Autodesk Inventor part; units mm, degrees
(part 2 of 3)
sketch "スケッチ2" plane through (0, 0, 4) normal (0, 0, 1) x (1, 0, 0)
  arc A0 (149.035, 132.768) -> (148.9038, 132.247) centre (154.985, 130.9929) ccw projected
  arc A1 (148.9038, 132.247) -> (148.0962, 132.247) centre (148.5, 105) ccw projected
  arc A2 (148.0962, 132.247) -> (147.965, 132.768) centre (142.015, 130.9929) ccw projected
  arc A3 (147.965, 132.768) -> (147.7093, 133.5027) centre (139.7412, 130.3182) ccw projected
  arc A4 (147.7093, 133.5027) -> (147.2659, 134.4742) centre (137.4161, 129.3913) ccw projected
  arc A5 (147.2659, 134.4742) -> (146.4842, 134.431) centre (148.5, 105) ccw projected
  arc A6 (146.4842, 134.431) -> (146.1503, 133.4167) centre (156.8334, 130.4626) ccw projected
  arc A7 (146.1503, 133.4167) -> (145.977, 132.6583) centre (154.4205, 131.128) ccw projected
  arc A8 (145.977, 132.6583) -> (145.904, 132.1261) centre (152.0862, 131.5485) ccw projected
  arc A9 (145.904, 132.1261) -> (145.1012, 132.0372) centre (148.5, 105) ccw projected
  arc A10 (145.1012, 132.0372) -> (144.9135, 132.5406) centre (139.195, 130.1217) ccw projected
  arc A11 (144.9135, 132.5406) -> (144.5786, 133.2427) centre (137.0091, 129.201) ccw projected
  arc A12 (144.5786, 133.2427) -> (144.031, 134.1595) centre (134.8001, 128.024) ccw projected
  arc A13 (144.031, 134.1595) -> (143.2588, 134.0307) centre (148.5, 105) ccw projected
  arc A14 (143.2588, 134.0307) -> (143.0385, 132.9857) centre (153.9817, 131.2248) ccw projected
  arc A15 (143.0385, 132.9857) -> (142.9497, 132.2129) centre (151.5102, 131.6208) ccw projected
  arc A16 (142.9497, 132.2129) -> (142.9356, 131.6758) centre (149.1439, 131.7819) ccw projected
  arc A17 (142.9356, 131.6758) -> (142.1475, 131.4992) centre (148.5, 105) ccw projected
  arc A18 (142.1475, 131.4992) -> (141.9056, 131.9789) centre (136.4879, 128.9456) ccw projected
  arc A19 (141.9056, 131.9789) -> (141.4955, 132.6399) centre (134.4166, 127.79) ccw projected
  arc A20 (141.4955, 132.6399) -> (140.8503, 133.4909) centre (132.3504, 126.3771) ccw projected
  arc A21 (140.8503, 133.4909) -> (140.097, 133.2779) centre (148.5, 105) ccw projected
  arc A22 (140.097, 133.2779) -> (139.993, 132.2151) centre (151.0635, 131.6687) ccw projected
  arc A23 (139.993, 132.2151) -> (139.9898, 131.4372) centre (148.5635, 131.7903) ccw projected
  arc A24 (139.9898, 131.4372) -> (140.0349, 130.9018) centre (146.1937, 131.6901) ccw projected
  arc A25 (140.0349, 130.9018) -> (139.271, 130.6396) centre (148.5, 105) ccw projected
  arc A26 (139.271, 130.6396) -> (138.9777, 131.0897) centre (133.9266, 127.4788) ccw projected
  arc A27 (138.9777, 131.0897) -> (138.4974, 131.7016) centre (131.995, 126.1024) ccw projected
  arc A28 (138.4974, 131.7016) -> (137.7625, 132.4765) centre (130.0968, 124.4708) ccw projected
  arc A29 (137.7625, 132.4765) -> (137.0372, 132.1819) centre (148.5, 105) ccw projected
  arc A30 (137.0372, 132.1819) -> (137.0508, 131.1141) centre (148.1142, 131.7888) ccw projected
  arc A31 (137.0508, 131.1141) -> (137.1331, 130.3405) centre (145.6159, 131.6347) ccw projected
  arc A32 (137.1331, 130.3405) -> (137.2368, 129.8134) centre (143.2716, 131.2744) ccw projected
  arc A33 (137.2368, 129.8134) -> (136.5064, 129.4687) centre (148.5, 105) ccw projected
  arc A34 (136.5064, 129.4687) -> (136.1654, 129.8839) centre (131.5421, 125.7392) ccw projected
  arc A35 (136.1654, 129.8839) -> (135.6207, 130.4392) centre (129.7737, 124.1586) ccw projected
  arc A36 (135.6207, 130.4392) -> (134.8051, 131.1285) centre (128.0665, 122.3281) ccw projected
  arc A37 (134.8051, 131.1285) -> (134.1165, 130.7559) centre (148.5, 105) ccw projected
  arc A38 (134.1165, 130.7559) -> (134.2475, 129.6961) centre (145.1695, 131.5838) ccw projected
  arc A39 (134.2475, 129.6961) -> (134.4144, 128.9363) centre (142.7034, 131.1558) ccw projected
  arc A40 (134.4144, 128.9363) -> (134.5755, 128.4237) centre (140.4129, 130.5398) ccw projected
  arc A41 (134.5755, 128.4237) -> (133.8875, 128.0008) centre (148.5, 105) ccw projected
  arc A42 (133.8875, 128.0008) -> (133.5029, 128.3759) centre (129.3636, 123.7478) ccw projected
  arc A43 (133.5029, 128.3759) -> (132.9003, 128.868) centre (127.7797, 121.9823) ccw projected
  arc A44 (132.9003, 128.868) -> (132.0138, 129.4634) centre (126.2843, 119.9751) ccw projected
  arc A45 (132.0138, 129.4634) -> (131.3705, 129.0173) centre (148.5, 105) ccw projected
  arc A46 (131.3705, 129.0173) -> (131.6172, 127.9783) centre (142.2653, 131.0561) ccw projected
  arc A47 (131.6172, 127.9783) -> (131.8667, 127.2415) centre (139.8612, 130.3594) ccw projected
  arc A48 (131.8667, 127.2415) -> (132.0832, 126.7498) centre (137.6524, 129.4952) ccw projected
  arc A49 (132.0832, 126.7498) -> (131.4459, 126.2537) centre (148.5, 105) ccw projected
  arc A50 (131.4459, 126.2537) -> (131.0223, 126.5843) centre (127.4173, 121.5289) ccw projected
  arc A51 (131.0223, 126.5843) -> (130.3693, 127.007) centre (126.0373, 119.5998) ccw projected
  arc A52 (130.3693, 127.007) -> (129.4227, 127.5013) centre (124.7718, 117.4403) ccw projected
  arc A53 (129.4227, 127.5013) -> (128.8323, 126.9871) centre (148.5, 105) ccw projected
  arc A54 (128.8323, 126.9871) -> (129.1919, 125.9816) centre (139.4368, 130.2121) ccw projected
  arc A55 (129.1919, 125.9816) -> (129.5209, 125.2767) centre (137.1239, 129.2551) ccw projected
  arc A56 (129.5209, 125.2767) -> (129.7902, 124.8118) centre (135.0236, 128.1532) ccw projected
  arc A57 (129.7902, 124.8118) -> (129.2113, 124.2486) centre (148.5, 105) ccw projected
  arc A58 (129.2113, 124.2486) -> (128.754, 124.5306) centre (125.727, 119.1093) ccw projected
  arc A59 (128.754, 124.5306) -> (128.0584, 124.8789) centre (124.5675, 117.0401) ccw projected
  arc A60 (128.0584, 124.8789) -> (127.0632, 125.2661) centre (123.5472, 114.7545) ccw projected
  arc A61 (127.0632, 125.2661) -> (126.5329, 124.69) centre (148.5, 105) ccw projected
  arc A62 (126.5329, 124.69) -> (127.0009, 123.7302) centre (136.7182, 129.062) ccw projected
  arc A63 (127.0009, 123.7302) -> (127.4055, 123.0658) centre (134.5247, 127.8564) ccw projected
  arc A64 (127.4055, 123.0658) -> (127.7243, 122.6333) centre (132.5583, 126.5301) ccw projected
  arc A65 (127.7243, 122.6333) -> (127.2109, 122.0099) centre (148.5, 105) ccw projected
  arc A66 (127.2109, 122.0099) -> (126.7253, 122.2398) centre (124.313, 116.5184) ccw projected
  arc A67 (126.7253, 122.2398) -> (125.9956, 122.5095) centre (123.3883, 114.3343) ccw projected
  arc A68 (125.9956, 122.5095) -> (124.9639, 122.7848) centre (122.6256, 111.9503) ccw projected
  arc A69 (124.9639, 122.7848) -> (124.5002, 122.154) centre (148.5, 105) ccw projected
  arc A70 (124.5002, 122.154) -> (125.0709, 121.2514) centre (134.1427, 127.6199) ccw projected
  arc A71 (125.0709, 121.2514) -> (125.5462, 120.6355) centre (132.0951, 126.1803) ccw projected
  arc A72 (125.5462, 120.6355) -> (125.9106, 120.2408) centre (130.2866, 124.6457) ccw projected
  arc A73 (125.9106, 120.2408) -> (125.4688, 119.5646) centre (148.5, 105) ccw projected
  arc A74 (125.4688, 119.5646) -> (124.9609, 119.7398) centre (123.1927, 113.7878) ccw projected
  arc A75 (124.9609, 119.7398) -> (124.206, 119.9276) centre (122.5139, 111.5151) ccw projected
  arc A76 (124.206, 119.9276) -> (123.1502, 120.0877) centre (122.0181, 109.0617) ccw projected
  arc A77 (123.1502, 120.0877) -> (122.7588, 119.4097) centre (148.5, 105) ccw projected
  arc A78 (122.7588, 119.4097) -> (123.4253, 118.5754) centre (131.7415, 125.9032) ccw projected
  arc A79 (123.4253, 118.5754) -> (123.9655, 118.0155) centre (129.8647, 124.2471) ccw projected
  arc A80 (123.9655, 118.0155) -> (124.3711, 117.6632) centre (128.2359, 122.5229) ccw projected
  arc A81 (124.3711, 117.6632) -> (124.0064, 116.9426) centre (148.5, 105) ccw projected
  arc A82 (124.0064, 116.9426) -> (123.4823, 117.0608) centre (122.3796, 110.9504) ccw projected
  arc A83 (123.4823, 117.0608) -> (122.7113, 117.1645) centre (121.9549, 108.6169) ccw projected
  arc A84 (122.7113, 117.1645) -> (121.6443, 117.2075) centre (121.732, 106.1238) ccw projected
  arc A85 (121.6443, 117.2075) -> (121.3298, 116.4905) centre (148.5, 105) ccw projected
  arc A86 (121.3298, 116.4905) -> (122.0841, 115.7346) centre (129.5437, 123.9327) ccw projected
  arc A87 (122.0841, 115.7346) -> (122.6825, 115.2375) centre (127.8604, 122.0802) ccw projected
  arc A88 (122.6825, 115.2375) -> (123.1245, 114.932) centre (126.4313, 120.1873) ccw projected
  arc A89 (123.1245, 114.932) -> (122.8413, 114.1756) centre (148.5, 105) ccw projected
  arc A90 (122.8413, 114.1756) -> (122.3074, 114.2355) centre (121.8835, 108.0408) ccw projected
  arc A91 (122.3074, 114.2355) -> (121.5297, 114.2537) centre (121.7181, 105.6748) ccw projected
  arc A92 (121.5297, 114.2537) -> (120.4644, 114.179) centre (121.7708, 103.1723) ccw projected
  arc A93 (120.4644, 114.179) -> (120.2307, 113.4318) centre (148.5, 105) ccw projected
  arc A94 (120.2307, 113.4318) -> (121.0636, 112.7635) centre (127.576, 121.7325) ccw projected
  arc A95 (121.0636, 112.7635) -> (121.713, 112.3353) centre (126.1067, 119.7061) ccw projected
  arc A96 (121.713, 112.3353) -> (122.1859, 112.0802) centre (124.8945, 117.6674) ccw projected
  arc A97 (122.1859, 112.0802) -> (121.9876, 111.2973) centre (148.5, 105) ccw projected
  arc A98 (121.9876, 111.2973) -> (121.4504, 111.298) centre (121.7106, 105.0943) ccw projected
  arc A99 (121.4504, 111.298) -> (120.6754, 111.2305) centre (121.8064, 102.7244) ccw projected
  arc A100 (120.6754, 111.2305) -> (119.6248, 111.0392) centre (122.1341, 100.243) ccw projected
  arc A101 (119.6248, 111.0392) -> (119.4747, 110.2708) centre (148.5, 105) ccw projected
  arc A102 (119.4747, 110.2708) -> (120.376, 109.6981) centre (125.8623, 119.3291) ccw projected
  arc A103 (120.376, 109.6981) -> (121.0687, 109.344) centre (124.6249, 117.1534) ccw projected
  arc A104 (121.0687, 109.344) -> (121.5667, 109.1425) centre (123.6442, 114.9937) ccw projected
  arc A105 (121.5667, 109.1425) -> (121.4558, 108.3425) centre (148.5, 105) ccw projected
  arc A106 (121.4558, 108.3425) -> (120.9217, 108.2841) centre (121.8628, 102.1467) ccw projected
  arc A107 (120.9217, 108.2841) -> (120.1588, 108.1318) centre (122.2187, 99.8017) ccw projected
  arc A108 (120.1588, 108.1318) -> (119.1357, 107.826) centre (122.8174, 97.3714) ccw projected
  arc A109 (119.1357, 107.826) -> (119.071, 107.0458) centre (148.5, 105) ccw projected
  arc A110 (119.071, 107.0458) -> (120.0299, 106.5757) centre (124.4233, 116.7518) ccw projected
  arc A111 (120.0299, 106.5757) -> (120.7573, 106.2999) centre (123.4328, 114.4531) ccw projected
  arc A112 (120.7573, 106.2999) -> (121.2745, 106.1544) centre (122.6957, 112.1987) ccw projected
  arc A113 (121.2745, 106.1544) -> (121.2522, 105.3471) centre (148.5, 105) ccw projected
  arc A114 (121.2522, 105.3471) -> (120.7278, 105.2303) centre (122.3383, 99.2337) ccw projected
  arc A115 (120.7278, 105.2303) -> (119.9863, 104.995) centre (122.9501, 96.9421) ccw projected
  arc A116 (119.9863, 104.995) -> (119.003, 104.5785) centre (123.8125, 94.5924) ccw projected
  arc A117 (119.003, 104.5785) -> (119.0246, 103.7959) centre (148.5, 105) ccw projected
  arc A118 (119.0246, 103.7959) -> (120.0294, 103.4342) centre (123.2767, 114.0318) ccw projected
  arc A119 (120.0294, 103.4342) -> (120.7827, 103.2401) centre (122.545, 111.6382) ccw projected
  arc A120 (120.7827, 103.2401) -> (121.3127, 103.1524) centre (122.0604, 109.3163) ccw projected
  arc A121 (121.3127, 103.1524) -> (121.3794, 102.3475) centre (148.5, 105) ccw projected
  arc A122 (121.3794, 102.3475) -> (120.871, 102.1738) centre (123.1315, 96.3907) ccw projected
  arc A123 (120.871, 102.1738) -> (120.1599, 101.8583) centre (123.9916, 94.1803) ccw projected
  arc A124 (120.1599, 101.8583) -> (119.2284, 101.3362) centre (125.1073, 91.9397) ccw projected
  arc A125 (119.2284, 101.3362) -> (119.3359, 100.5607) centre (148.5, 105) ccw projected
  arc A126 (119.3359, 100.5607) -> (120.3744, 100.3117) centre (122.4362, 111.2023) ccw projected
  arc A127 (120.3744, 100.3117) -> (121.1445, 100.2017) centre (121.9723, 108.7426) ccw projected
  arc A128 (121.1445, 100.2017) -> (121.681, 100.1728) centre (121.746, 106.3816) ccw projected
  arc A129 (121.681, 100.1728) -> (121.8358, 99.3801) centre (148.5, 105) ccw projected
  arc A130 (121.8358, 99.3801) -> (121.3496, 99.1515) centre (124.2325, 93.6522) ccw projected
  arc A131 (121.3496, 99.1515) -> (120.6776, 98.7597) centre (125.3306, 91.5499) ccw projected
  arc A132 (120.6776, 98.7597) -> (119.8091, 98.1383) centre (126.686, 89.4456) ccw projected
  arc A133 (119.8091, 98.1383) -> (120.0013, 97.3793) centre (148.5, 105) ccw projected
  arc A134 (120.0013, 97.3793) -> (121.0608, 97.2461) centre (121.9121, 108.2974) ccw projected
  arc A135 (121.0608, 97.2461) -> (121.8384, 97.2214) centre (121.7216, 105.8016) ccw projected
  arc A136 (121.8384, 97.2214) -> (122.3748, 97.2518) centre (121.7564, 103.43) ccw projected
  arc A137 (122.3748, 97.2518) -> (122.6159, 96.481) centre (148.5, 105) ccw projected
  arc A138 (122.6159, 96.481) -> (122.1578, 96.2002) centre (125.6281, 91.0515) ccw projected
  arc A139 (122.1578, 96.2002) -> (121.5329, 95.7369) centre (126.9509, 89.0827) ccw projected
  arc A140 (121.5329, 95.7369) -> (120.7381, 95.0237) centre (128.5295, 87.1403) ccw projected
  arc A141 (120.7381, 95.0237) -> (121.0126, 94.2905) centre (148.5, 105) ccw projected
  arc A142 (121.0126, 94.2905) -> (122.0804, 94.2747) centre (121.7107, 105.3525) ccw projected
  arc A143 (122.0804, 94.2747) -> (122.8559, 94.3357) centre (121.7959, 102.8509) ccw projected
  arc A144 (122.8559, 94.3357) -> (123.3857, 94.4248) centre (122.0915, 100.4975) ccw projected
  arc A145 (123.3857, 94.4248) -> (123.7101, 93.6852) centre (148.5, 105) ccw projected
  arc A146 (123.7101, 93.6852) -> (123.2857, 93.3558) centre (127.3014, 88.62) ccw projected
  arc A147 (123.2857, 93.3558) -> (122.7156, 92.8265) centre (128.8327, 86.8087) ccw projected
  arc A148 (122.7156, 92.8265) -> (122.0041, 92.0302) centre (130.6154, 85.0518) ccw projected
  arc A149 (122.0041, 92.0302) -> (122.3576, 91.3317) centre (148.5, 105) ccw projected
  arc A150 (122.3576, 91.3317) -> (123.4206, 91.4334) centre (121.8345, 102.4033) ccw projected
  arc A151 (123.4206, 91.4334) -> (124.1847, 91.5793) centre (122.1944, 99.9263) ccw projected
  arc A152 (124.1847, 91.5793) -> (124.7015, 91.7262) centre (122.7471, 97.6197) ccw projected
  arc A153 (124.7015, 91.7262) -> (125.1053, 91.0268) centre (148.5, 105) ccw projected
  arc A154 (125.1053, 91.0268) -> (124.7197, 90.6527) centre (129.232, 86.3874) ccw projected
  arc A155 (124.7197, 90.6527) -> (124.2113, 90.0639) centre (130.9532, 84.7555) ccw projected
  arc A156 (124.2113, 90.0639) -> (123.5917, 89.1942) centre (132.9185, 83.2054) ccw projected
  arc A157 (123.5917, 89.1942) -> (124.0199, 88.5387) centre (148.5, 105) ccw projected
  arc A158 (124.0199, 88.5387) -> (125.0653, 88.7568) centre (122.282, 99.4856) ccw projected
  arc A159 (125.0653, 88.7568) -> (125.8087, 88.9859) centre (122.9122, 97.0632) ccw projected
  arc A160 (125.8087, 88.9859) -> (126.3062, 89.1887) centre (123.7152, 94.8315) ccw projected
  arc A161 (126.3062, 89.1887) -> (126.7845, 88.538) centre (148.5, 105) ccw projected
  arc A162 (126.7845, 88.538) -> (126.4424, 88.1237) centre (131.3965, 84.3808) ccw projected
  arc A163 (126.4424, 88.1237) -> (126.0018, 87.4826) centre (133.2868, 82.9481) ccw projected
  arc A164 (126.0018, 87.4826) -> (125.4816, 86.55) centre (135.4106, 81.6236) ccw projected
  arc A165 (125.4816, 86.55) -> (125.9793, 85.9456) centre (148.5, 105) ccw projected
  arc A166 (125.9793, 85.9456) -> (126.9944, 86.2773) centre (123.0478, 96.6349) ccw projected
  arc A167 (126.9944, 86.2773) -> (127.7081, 86.5869) centre (123.9406, 94.2966) ccw projected
  arc A168 (127.7081, 86.5869) -> (128.1802, 86.8432) centre (124.9843, 92.1667) ccw projected
  arc A169 (128.1802, 86.8432) -> (128.7272, 86.249) centre (148.5, 105) ccw projected
  arc A170 (128.7272, 86.249) -> (128.4328, 85.7996) centre (133.7686, 82.6244) ccw projected
  arc A171 (128.4328, 85.7996) -> (128.0654, 85.1139) centre (135.805, 81.4084) ccw projected
  arc A172 (128.0654, 85.1139) -> (127.651, 84.1297) centre (138.0617, 80.3255) ccw projected
  arc A173 (127.651, 84.1297) -> (128.2121, 83.5838) centre (148.5, 105) ccw projected
  arc A174 (128.2121, 83.5838) -> (129.1845, 84.0252) centre (124.1225, 93.8857) ccw projected
  arc A175 (129.1845, 84.0252) -> (129.8599, 84.4113) centre (125.2672, 91.6598) ccw projected
  arc A176 (129.8599, 84.4113) -> (130.3009, 84.7181) centre (126.5388, 89.6576) ccw projected
  arc A177 (130.3009, 84.7181) -> (130.91, 84.1876) centre (148.5, 105) ccw projected
  arc A178 (130.91, 84.1876) -> (130.6668, 83.7086) centre (136.3195, 81.1396) ccw projected
  arc A179 (130.6668, 83.7086) -> (130.377, 82.9867) centre (138.4773, 80.155) ccw projected
  arc A180 (130.377, 82.9867) -> (130.0734, 81.9628) centre (140.8394, 79.3269) ccw projected
  arc A181 (130.0734, 81.9628) -> (130.6912, 81.482) centre (148.5, 105) ccw projected
  arc A182 (130.6912, 81.482) -> (131.6092, 82.0276) centre (125.4931, 91.2715) ccw projected
  arc A183 (131.6092, 82.0276) -> (132.2379, 82.4857) centre (126.8757, 89.1849) ccw projected
  arc A184 (132.2379, 82.4857) -> (132.6426, 82.8391) centre (128.3599, 87.3348) ccw projected
  arc A185 (132.6426, 82.8391) -> (133.3063, 82.3789) centre (148.5, 105) ccw projected
  arc A186 (133.3063, 82.3789) -> (133.1172, 81.876) centre (139.0183, 79.9445) ccw projected
  arc A187 (133.1172, 81.876) -> (132.9087, 81.1266) centre (141.2713, 79.2032) ccw projected
  arc A188 (132.9087, 81.1266) -> (132.7195, 80.0756) centre (143.7101, 78.64) ccw projected
  arc A189 (132.7195, 80.0756) -> (133.3865, 79.6656) centre (148.5, 105) ccw projected
  arc A190 (133.3865, 79.6656) -> (134.2388, 80.3089) centre (127.143, 88.8238) ccw projected
  arc A191 (134.2388, 80.3089) -> (134.8134, 80.8334) centre (128.7467, 86.9021) ccw projected
  arc A192 (134.8134, 80.8334) -> (135.1767, 81.2292) centre (130.4254, 85.2265) ccw projected
  arc A193 (135.1767, 81.2292) -> (135.887, 80.8448) centre (148.5, 105) ccw projected
  arc A194 (135.887, 80.8448) -> (135.7544, 80.3241) centre (141.8321, 79.0535) ccw projected
  arc A195 (135.7544, 80.3241) -> (135.6296, 79.5563) centre (144.153, 78.5646) ccw projected
  arc A196 (135.6296, 79.5563) -> (135.5572, 78.4909) centre (146.639, 78.2731) ccw projected
  arc A197 (135.5572, 78.4909) -> (136.2652, 78.1567) centre (148.5, 105) ccw projected
  arc A198 (136.2652, 78.1567) -> (137.0416, 78.8899) centre (129.0521, 86.5726) ccw projected
  arc A199 (137.0416, 78.8899) -> (137.555, 79.4744) centre (130.8575, 84.8389) ccw projected
  arc A200 (137.555, 79.4744) -> (137.8726, 79.9078) centre (132.7104, 83.3581) ccw projected
  arc A201 (137.8726, 79.9078) -> (138.6208, 79.6038) centre (148.5, 105) ccw projected
  arc A202 (138.6208, 79.6038) -> (138.5463, 79.0718) centre (144.7269, 78.4774) ccw projected
  arc A203 (138.5463, 79.0718) -> (138.5067, 78.2949) centre (147.0875, 78.2468) ccw projected
  arc A204 (138.5067, 78.2949) -> (138.552, 77.228) centre (149.5905, 78.2306) ccw projected
  arc A205 (138.552, 77.228) -> (139.2925, 76.9737) centre (148.5, 105) ccw projected
  arc A206 (139.2925, 76.9737) -> (139.9835, 77.7879) centre (131.1973, 84.545) ccw projected
  arc A207 (139.9835, 77.7879) -> (140.4294, 78.4253) centre (133.1825, 83.0204) ccw projected
  arc A208 (140.4294, 78.4253) -> (140.6974, 78.891) centre (135.187, 81.7525) ccw projected
  arc A209 (140.6974, 78.891) -> (141.4746, 78.6712) centre (148.5, 105) ccw projected
  arc A210 (141.4746, 78.6712) -> (141.459, 78.1342) centre (147.6675, 78.2233) ccw projected
  arc A211 (141.459, 78.1342) -> (141.5051, 77.3576) centre (150.0392, 78.2538) ccw projected
  arc A212 (141.5051, 77.3576) -> (141.6675, 76.3021) centre (152.5287, 78.513) ccw projected
  arc A213 (141.6675, 76.3021) -> (142.4315, 76.1309) centre (148.5, 105) ccw projected
  arc A214 (142.4315, 76.1309) -> (143.0287, 77.0162) centre (133.5526, 82.7657) ccw projected
  arc A215 (143.0287, 77.0162) -> (143.4018, 77.6988) centre (135.6934, 81.4688) ccw projected
  arc A216 (143.4018, 77.6988) -> (143.617, 78.1911) centre (137.8252, 80.429) ccw projected
  arc A217 (143.617, 78.1911) -> (144.4136, 78.0581) centre (148.5, 105) ccw projected
  arc A218 (144.4136, 78.0581) -> (144.4572, 77.5227) centre (150.6182, 78.2943) ccw projected
  arc A219 (144.4572, 77.5227) -> (144.5885, 76.7559) centre (152.9721, 78.5855) ccw projected
  arc A220 (144.5885, 76.7559) -> (144.866, 75.7247) centre (155.4181, 79.117) ccw projected
  arc A221 (144.866, 75.7247) -> (145.6441, 75.6386) centre (148.5, 105) ccw projected
  arc A222 (145.6441, 75.6386) -> (146.1404, 76.5841) centre (136.0892, 81.2563) ccw projected
  arc A223 (146.1404, 76.5841) -> (146.4361, 77.3036) centre (138.3598, 80.2028) ccw projected
  arc A224 (146.4361, 77.3036) -> (146.5958, 77.8166) centre (140.593, 79.4039) ccw projected
  arc A225 (146.5958, 77.8166) -> (147.4022, 77.7721) centre (148.5, 105) ccw projected
  arc A226 (147.4022, 77.7721) -> (147.5045, 77.2447) centre (153.5432, 78.6894) ccw projected
  arc A227 (147.5045, 77.2447) -> (147.7193, 76.497) centre (155.8508, 79.2378) ccw projected
  arc A228 (147.7193, 76.497) -> (148.1085, 75.5026) centre (158.2234, 80.0351) ccw projected
  arc A229 (148.1085, 75.5026) -> (148.8915, 75.5026) centre (148.5, 105) ccw projected
  arc A230 (148.8915, 75.5026) -> (149.2807, 76.497) centre (138.7766, 80.0351) ccw projected
  arc A231 (149.2807, 76.497) -> (149.4955, 77.2447) centre (141.1492, 79.2378) ccw projected
  arc A232 (149.4955, 77.2447) -> (149.5978, 77.7721) centre (143.4568, 78.6894) ccw projected
  arc A233 (149.5978, 77.7721) -> (150.4042, 77.8166) centre (148.5, 105) ccw projected
  arc A234 (150.4042, 77.8166) -> (150.5639, 77.3036) centre (156.407, 79.4039) ccw projected
  arc A235 (150.5639, 77.3036) -> (150.8596, 76.5841) centre (158.6402, 80.2028) ccw projected
  arc A236 (150.8596, 76.5841) -> (151.3559, 75.6386) centre (160.9108, 81.2563) ccw projected
  arc A237 (151.3559, 75.6386) -> (152.134, 75.7247) centre (148.5, 105) ccw projected
  arc A238 (152.134, 75.7247) -> (152.4115, 76.7559) centre (141.5819, 79.117) ccw projected
  arc A239 (152.4115, 76.7559) -> (152.5428, 77.5227) centre (144.0279, 78.5855) ccw projected
  arc A240 (152.5428, 77.5227) -> (152.5864, 78.0581) centre (146.3818, 78.2943) ccw projected
  arc A241 (152.5864, 78.0581) -> (153.383, 78.1911) centre (148.5, 105) ccw projected
  arc A242 (153.383, 78.1911) -> (153.5982, 77.6988) centre (159.1748, 80.429) ccw projected
  arc A243 (153.5982, 77.6988) -> (153.9713, 77.0162) centre (161.3066, 81.4688) ccw projected
  arc A244 (153.9713, 77.0162) -> (154.5685, 76.1309) centre (163.4474, 82.7657) ccw projected
  arc A245 (154.5685, 76.1309) -> (155.3325, 76.3021) centre (148.5, 105) ccw projected
  arc A246 (155.3325, 76.3021) -> (155.4949, 77.3576) centre (144.4713, 78.513) ccw projected
  arc A247 (155.4949, 77.3576) -> (155.541, 78.1342) centre (146.9608, 78.2538) ccw projected
  arc A248 (155.541, 78.1342) -> (155.5254, 78.6712) centre (149.3325, 78.2233) ccw projected
  arc A249 (155.5254, 78.6712) -> (156.3026, 78.891) centre (148.5, 105) ccw projected
  arc A250 (156.3026, 78.891) -> (156.5706, 78.4253) centre (161.813, 81.7525) ccw projected
  arc A251 (156.5706, 78.4253) -> (157.0165, 77.7879) centre (163.8175, 83.0204) ccw projected
  arc A252 (157.0165, 77.7879) -> (157.7075, 76.9737) centre (165.8027, 84.545) ccw projected
  arc A253 (157.7075, 76.9737) -> (158.448, 77.228) centre (148.5, 105) ccw projected
  arc A254 (158.448, 77.228) -> (158.4933, 78.2949) centre (147.4095, 78.2306) ccw projected
  arc A255 (158.4933, 78.2949) -> (158.4537, 79.0718) centre (149.9125, 78.2468) ccw projected
  arc A256 (158.4537, 79.0718) -> (158.3792, 79.6038) centre (152.2731, 78.4774) ccw projected
  arc A257 (158.3792, 79.6038) -> (159.1274, 79.9078) centre (148.5, 105) ccw projected
  arc A258 (159.1274, 79.9078) -> (159.445, 79.4744) centre (164.2896, 83.3581) ccw projected
  arc A259 (159.445, 79.4744) -> (159.9584, 78.8899) centre (166.1425, 84.8389) ccw projected
  arc A260 (159.9584, 78.8899) -> (160.7348, 78.1567) centre (167.9479, 86.5726) ccw projected
  arc A261 (160.7348, 78.1567) -> (161.4428, 78.4909) centre (148.5, 105) ccw projected
  arc A262 (161.4428, 78.4909) -> (161.3704, 79.5563) centre (150.361, 78.2731) ccw projected
  arc A263 (161.3704, 79.5563) -> (161.2456, 80.3241) centre (152.847, 78.5646) ccw projected
  arc A264 (161.2456, 80.3241) -> (161.113, 80.8448) centre (155.1679, 79.0535) ccw projected
  arc A265 (161.113, 80.8448) -> (161.8233, 81.2292) centre (148.5, 105) ccw projected
  arc A266 (161.8233, 81.2292) -> (162.1866, 80.8334) centre (166.5746, 85.2265) ccw projected
  arc A267 (162.1866, 80.8334) -> (162.7612, 80.3089) centre (168.2533, 86.9021) ccw projected
  arc A268 (162.7612, 80.3089) -> (163.6135, 79.6656) centre (169.857, 88.8238) ccw projected
  arc A269 (163.6135, 79.6656) -> (164.2805, 80.0756) centre (148.5, 105) ccw projected
  arc A270 (164.2805, 80.0756) -> (164.0913, 81.1266) centre (153.2899, 78.64) ccw projected
  arc A271 (164.0913, 81.1266) -> (163.8828, 81.876) centre (155.7287, 79.2032) ccw projected
  arc A272 (163.8828, 81.876) -> (163.6937, 82.3789) centre (157.9817, 79.9445) ccw projected
  arc A273 (163.6937, 82.3789) -> (164.3574, 82.8391) centre (148.5, 105) ccw projected
  arc A274 (164.3574, 82.8391) -> (164.7621, 82.4857) centre (168.6401, 87.3348) ccw projected
  arc A275 (164.7621, 82.4857) -> (165.3908, 82.0276) centre (170.1243, 89.1849) ccw projected
  arc A276 (165.3908, 82.0276) -> (166.3088, 81.482) centre (171.5069, 91.2715) ccw projected
  arc A277 (166.3088, 81.482) -> (166.9266, 81.9628) centre (148.5, 105) ccw projected
  arc A278 (166.9266, 81.9628) -> (166.623, 82.9867) centre (156.1606, 79.3269) ccw projected
  arc A279 (166.623, 82.9867) -> (166.3332, 83.7086) centre (158.5227, 80.155) ccw projected
  arc A280 (166.3332, 83.7086) -> (166.09, 84.1876) centre (160.6805, 81.1396) ccw projected
  arc A281 (166.09, 84.1876) -> (166.6991, 84.7181) centre (148.5, 105) ccw projected
  arc A282 (166.6991, 84.7181) -> (167.1401, 84.4113) centre (170.4612, 89.6576) ccw projected
  arc A283 (167.1401, 84.4113) -> (167.8155, 84.0252) centre (171.7328, 91.6598) ccw projected
  arc A284 (167.8155, 84.0252) -> (168.7879, 83.5838) centre (172.8775, 93.8857) ccw projected
  arc A285 (168.7879, 83.5838) -> (169.349, 84.1297) centre (148.5, 105) ccw projected
  arc A286 (169.349, 84.1297) -> (168.9346, 85.1139) centre (158.9383, 80.3255) ccw projected
  arc A287 (168.9346, 85.1139) -> (168.5672, 85.7996) centre (161.195, 81.4084) ccw projected
  arc A288 (168.5672, 85.7996) -> (168.2728, 86.249) centre (163.2314, 82.6244) ccw projected
  arc A289 (168.2728, 86.249) -> (168.8198, 86.8432) centre (148.5, 105) ccw projected
  arc A290 (168.8198, 86.8432) -> (169.2919, 86.5869) centre (172.0157, 92.1667) ccw projected
  arc A291 (169.2919, 86.5869) -> (170.0056, 86.2773) centre (173.0594, 94.2966) ccw projected
  arc A292 (170.0056, 86.2773) -> (171.0207, 85.9456) centre (173.9522, 96.6349) ccw projected
  arc A293 (171.0207, 85.9456) -> (171.5184, 86.55) centre (148.5, 105) ccw projected
  arc A294 (171.5184, 86.55) -> (170.9982, 87.4826) centre (161.5894, 81.6236) ccw projected
  arc A295 (170.9982, 87.4826) -> (170.5576, 88.1237) centre (163.7132, 82.9481) ccw projected
  arc A296 (170.5576, 88.1237) -> (170.2155, 88.538) centre (165.6035, 84.3808) ccw projected
  arc A297 (170.2155, 88.538) -> (170.6938, 89.1887) centre (148.5, 105) ccw projected
  arc A298 (170.6938, 89.1887) -> (171.1913, 88.9859) centre (173.2848, 94.8315) ccw projected
  arc A299 (171.1913, 88.9859) -> (171.9347, 88.7568) centre (174.0878, 97.0632) ccw projected
  arc A300 (171.9347, 88.7568) -> (172.9801, 88.5387) centre (174.718, 99.4856) ccw projected
  arc A301 (172.9801, 88.5387) -> (173.4083, 89.1942) centre (148.5, 105) ccw projected
  arc A302 (173.4083, 89.1942) -> (172.7887, 90.0639) centre (164.0815, 83.2054) ccw projected
  arc A303 (172.7887, 90.0639) -> (172.2803, 90.6527) centre (166.0468, 84.7555) ccw projected
  arc A304 (172.2803, 90.6527) -> (171.8947, 91.0268) centre (167.768, 86.3874) ccw projected
  arc A305 (171.8947, 91.0268) -> (172.2985, 91.7262) centre (148.5, 105) ccw projected
  arc A306 (172.2985, 91.7262) -> (172.8153, 91.5793) centre (174.2529, 97.6197) ccw projected
  arc A307 (172.8153, 91.5793) -> (173.5794, 91.4334) centre (174.8056, 99.9263) ccw projected
  arc A308 (173.5794, 91.4334) -> (174.6424, 91.3317) centre (175.1655, 102.4033) ccw projected
  arc A309 (174.6424, 91.3317) -> (174.9959, 92.0302) centre (148.5, 105) ccw projected
  arc A310 (174.9959, 92.0302) -> (174.2844, 92.8265) centre (166.3846, 85.0518) ccw projected
  arc A311 (174.2844, 92.8265) -> (173.7143, 93.3558) centre (168.1673, 86.8087) ccw projected
  arc A312 (173.7143, 93.3558) -> (173.2899, 93.6852) centre (169.6986, 88.62) ccw projected
  arc A313 (173.2899, 93.6852) -> (173.6143, 94.4248) centre (148.5, 105) ccw projected
  arc A314 (173.6143, 94.4248) -> (174.1441, 94.3357) centre (174.9085, 100.4975) ccw projected
  arc A315 (174.1441, 94.3357) -> (174.9196, 94.2747) centre (175.2041, 102.8509) ccw projected
  arc A316 (174.9196, 94.2747) -> (175.9874, 94.2905) centre (175.2893, 105.3525) ccw projected
  arc A317 (175.9874, 94.2905) -> (176.2619, 95.0237) centre (148.5, 105) ccw projected
  arc A318 (176.2619, 95.0237) -> (175.4671, 95.7369) centre (168.4705, 87.1403) ccw projected
  arc A319 (175.4671, 95.7369) -> (174.8422, 96.2002) centre (170.0491, 89.0827) ccw projected
  arc A320 (174.8422, 96.2002) -> (174.3841, 96.481) centre (171.3719, 91.0515) ccw projected
  arc A321 (174.3841, 96.481) -> (174.6252, 97.2518) centre (148.5, 105) ccw projected
  arc A322 (174.6252, 97.2518) -> (175.1616, 97.2214) centre (175.2436, 103.43) ccw projected
  arc A323 (175.1616, 97.2214) -> (175.9392, 97.2461) centre (175.2784, 105.8016) ccw projected
  arc A324 (175.9392, 97.2461) -> (176.9987, 97.3793) centre (175.0879, 108.2974) ccw projected
  arc A325 (176.9987, 97.3793) -> (177.1909, 98.1383) centre (148.5, 105) ccw projected
  arc A326 (177.1909, 98.1383) -> (176.3224, 98.7597) centre (170.314, 89.4456) ccw projected
  arc A327 (176.3224, 98.7597) -> (175.6504, 99.1515) centre (171.6694, 91.5499) ccw projected
  arc A328 (175.6504, 99.1515) -> (175.1642, 99.3801) centre (172.7675, 93.6522) ccw projected
  arc A329 (175.1642, 99.3801) -> (175.319, 100.1728) centre (148.5, 105) ccw projected
  arc A330 (175.319, 100.1728) -> (175.8555, 100.2017) centre (175.254, 106.3816) ccw projected
  arc A331 (175.8555, 100.2017) -> (176.6256, 100.3117) centre (175.0277, 108.7426) ccw projected
  arc A332 (176.6256, 100.3117) -> (177.6641, 100.5607) centre (174.5638, 111.2023) ccw projected
  arc A333 (177.6641, 100.5607) -> (177.7716, 101.3362) centre (148.5, 105) ccw projected
  arc A334 (177.7716, 101.3362) -> (176.8401, 101.8583) centre (171.8927, 91.9397) ccw projected
  arc A335 (176.8401, 101.8583) -> (176.129, 102.1738) centre (173.0084, 94.1803) ccw projected
  arc A336 (176.129, 102.1738) -> (175.6206, 102.3475) centre (173.8685, 96.3907) ccw projected
  arc A337 (175.6206, 102.3475) -> (175.6873, 103.1524) centre (148.5, 105) ccw projected
  arc A338 (175.6873, 103.1524) -> (176.2173, 103.2401) centre (174.9396, 109.3163) ccw projected
  arc A339 (176.2173, 103.2401) -> (176.9706, 103.4342) centre (174.455, 111.6382) ccw projected
  arc A340 (176.9706, 103.4342) -> (177.9754, 103.7959) centre (173.7233, 114.0318) ccw projected
  arc A341 (177.9754, 103.7959) -> (177.997, 104.5785) centre (148.5, 105) ccw projected
  arc A342 (177.997, 104.5785) -> (177.0137, 104.995) centre (173.1875, 94.5924) ccw projected
  arc A343 (177.0137, 104.995) -> (176.2722, 105.2303) centre (174.0499, 96.9421) ccw projected
  arc A344 (176.2722, 105.2303) -> (175.7478, 105.3471) centre (174.6617, 99.2337) ccw projected
  arc A345 (175.7478, 105.3471) -> (175.7255, 106.1544) centre (148.5, 105) ccw projected
  arc A346 (175.7255, 106.1544) -> (176.2427, 106.2999) centre (174.3043, 112.1987) ccw projected
  arc A347 (176.2427, 106.2999) -> (176.9701, 106.5757) centre (173.5672, 114.4531) ccw projected
  arc A348 (176.9701, 106.5757) -> (177.929, 107.0458) centre (172.5767, 116.7518) ccw projected
  arc A349 (177.929, 107.0458) -> (177.8643, 107.826) centre (148.5, 105) ccw projected
  arc A350 (177.8643, 107.826) -> (176.8412, 108.1318) centre (174.1826, 97.3714) ccw projected
  arc A351 (176.8412, 108.1318) -> (176.0783, 108.2841) centre (174.7813, 99.8017) ccw projected
  arc A352 (176.0783, 108.2841) -> (175.5442, 108.3425) centre (175.1372, 102.1467) ccw projected
  arc A353 (175.5442, 108.3425) -> (175.4333, 109.1425) centre (148.5, 105) ccw projected
  arc A354 (175.4333, 109.1425) -> (175.9313, 109.344) centre (173.3558, 114.9937) ccw projected
  arc A355 (175.9313, 109.344) -> (176.624, 109.6981) centre (172.3751, 117.1534) ccw projected
  arc A356 (176.624, 109.6981) -> (177.5253, 110.2708) centre (171.1377, 119.3291) ccw projected
  arc A357 (177.5253, 110.2708) -> (177.3752, 111.0392) centre (148.5, 105) ccw projected
  arc A358 (177.3752, 111.0392) -> (176.3246, 111.2305) centre (174.8659, 100.243) ccw projected
  arc A359 (176.3246, 111.2305) -> (175.5496, 111.298) centre (175.1936, 102.7244) ccw projected
  arc A360 (175.5496, 111.298) -> (175.0124, 111.2973) centre (175.2894, 105.0943) ccw projected
  arc A361 (175.0124, 111.2973) -> (174.8141, 112.0802) centre (148.5, 105) ccw projected
  arc A362 (174.8141, 112.0802) -> (175.287, 112.3353) centre (172.1055, 117.6674) ccw projected
  arc A363 (175.287, 112.3353) -> (175.9364, 112.7635) centre (170.8933, 119.7061) ccw projected
  arc A364 (175.9364, 112.7635) -> (176.7693, 113.4318) centre (169.424, 121.7325) ccw projected
  arc A365 (176.7693, 113.4318) -> (176.5356, 114.179) centre (148.5, 105) ccw projected
  arc A366 (176.5356, 114.179) -> (175.4703, 114.2537) centre (175.2292, 103.1723) ccw projected
  arc A367 (175.4703, 114.2537) -> (174.6926, 114.2355) centre (175.2819, 105.6748) ccw projected
  arc A368 (174.6926, 114.2355) -> (174.1587, 114.1756) centre (175.1165, 108.0408) ccw projected
  arc A369 (174.1587, 114.1756) -> (173.8755, 114.932) centre (148.5, 105) ccw projected
  arc A370 (173.8755, 114.932) -> (174.3175, 115.2375) centre (170.5687, 120.1873) ccw projected
  arc A371 (174.3175, 115.2375) -> (174.9159, 115.7346) centre (169.1396, 122.0802) ccw projected
  arc A372 (174.9159, 115.7346) -> (175.6702, 116.4905) centre (167.4563, 123.9327) ccw projected
  arc A373 (175.6702, 116.4905) -> (175.3557, 117.2075) centre (148.5, 105) ccw projected
  arc A374 (175.3557, 117.2075) -> (174.2887, 117.1645) centre (175.268, 106.1238) ccw projected
  arc A375 (174.2887, 117.1645) -> (173.5177, 117.0608) centre (175.0451, 108.6169) ccw projected
  arc A376 (173.5177, 117.0608) -> (172.9936, 116.9426) centre (174.6204, 110.9504) ccw projected
  arc A377 (172.9936, 116.9426) -> (172.6289, 117.6632) centre (148.5, 105) ccw projected
  arc A378 (172.6289, 117.6632) -> (173.0345, 118.0155) centre (168.7641, 122.5229) ccw projected
  arc A379 (173.0345, 118.0155) -> (173.5747, 118.5754) centre (167.1353, 124.2471) ccw projected
  arc A380 (173.5747, 118.5754) -> (174.2412, 119.4097) centre (165.2585, 125.9032) ccw projected
  arc A381 (174.2412, 119.4097) -> (173.8498, 120.0877) centre (148.5, 105) ccw projected
  arc A382 (173.8498, 120.0877) -> (172.794, 119.9276) centre (174.9819, 109.0617) ccw projected
  arc A383 (172.794, 119.9276) -> (172.0391, 119.7398) centre (174.4861, 111.5151) ccw projected
  arc A384 (172.0391, 119.7398) -> (171.5312, 119.5646) centre (173.8073, 113.7878) ccw projected
  arc A385 (171.5312, 119.5646) -> (171.0894, 120.2408) centre (148.5, 105) ccw projected
  arc A386 (171.0894, 120.2408) -> (171.4538, 120.6355) centre (166.7134, 124.6457) ccw projected
  arc A387 (171.4538, 120.6355) -> (171.9291, 121.2514) centre (164.9049, 126.1803) ccw projected
  arc A388 (171.9291, 121.2514) -> (172.4998, 122.154) centre (162.8573, 127.6199) ccw projected
  arc A389 (172.4998, 122.154) -> (172.0361, 122.7848) centre (148.5, 105) ccw projected
  arc A390 (172.0361, 122.7848) -> (171.0044, 122.5095) centre (174.3744, 111.9503) ccw projected
  arc A391 (171.0044, 122.5095) -> (170.2747, 122.2398) centre (173.6117, 114.3343) ccw projected
  arc A392 (170.2747, 122.2398) -> (169.7891, 122.0099) centre (172.687, 116.5184) ccw projected
  arc A393 (169.7891, 122.0099) -> (169.2757, 122.6333) centre (148.5, 105) ccw projected
  arc A394 (169.2757, 122.6333) -> (169.5945, 123.0658) centre (164.4417, 126.5301) ccw projected
  arc A395 (169.5945, 123.0658) -> (169.9991, 123.7302) centre (162.4753, 127.8564) ccw projected
  arc A396 (169.9991, 123.7302) -> (170.4671, 124.69) centre (160.2818, 129.062) ccw projected
  arc A397 (170.4671, 124.69) -> (169.9368, 125.2661) centre (148.5, 105) ccw projected
  arc A398 (169.9368, 125.2661) -> (168.9416, 124.8789) centre (173.4528, 114.7545) ccw projected
  arc A399 (168.9416, 124.8789) -> (168.246, 124.5306) centre (172.4325, 117.0401) ccw projected
  arc A400 (168.246, 124.5306) -> (167.7887, 124.2486) centre (171.273, 119.1093) ccw projected
  arc A401 (167.7887, 124.2486) -> (167.2098, 124.8118) centre (148.5, 105) ccw projected
  arc A402 (167.2098, 124.8118) -> (167.4791, 125.2767) centre (161.9764, 128.1532) ccw projected
  arc A403 (167.4791, 125.2767) -> (167.8081, 125.9816) centre (159.8761, 129.2551) ccw projected
  arc A404 (167.8081, 125.9816) -> (168.1677, 126.9871) centre (157.5632, 130.2121) ccw projected
  arc A405 (168.1677, 126.9871) -> (167.5773, 127.5013) centre (148.5, 105) ccw projected
  arc A406 (167.5773, 127.5013) -> (166.6307, 127.007) centre (172.2282, 117.4403) ccw projected
  arc A407 (166.6307, 127.007) -> (165.9777, 126.5843) centre (170.9627, 119.5998) ccw projected
  arc A408 (165.9777, 126.5843) -> (165.5541, 126.2537) centre (169.5827, 121.5289) ccw projected
  arc A409 (165.5541, 126.2537) -> (164.9168, 126.7498) centre (148.5, 105) ccw projected
  arc A410 (164.9168, 126.7498) -> (165.1333, 127.2415) centre (159.3476, 129.4952) ccw projected
  arc A411 (165.1333, 127.2415) -> (165.3828, 127.9783) centre (157.1388, 130.3594) ccw projected
  arc A412 (165.3828, 127.9783) -> (165.6295, 129.0173) centre (154.7347, 131.0561) ccw projected
  arc A413 (165.6295, 129.0173) -> (164.9862, 129.4634) centre (148.5, 105) ccw projected
  arc A414 (164.9862, 129.4634) -> (164.0997, 128.868) centre (170.7157, 119.9751) ccw projected
  arc A415 (164.0997, 128.868) -> (163.4971, 128.3759) centre (169.2203, 121.9823) ccw projected
  arc A416 (163.4971, 128.3759) -> (163.1125, 128.0008) centre (167.6364, 123.7478) ccw projected
  arc A417 (163.1125, 128.0008) -> (162.4245, 128.4237) centre (148.5, 105) ccw projected
  arc A418 (162.4245, 128.4237) -> (162.5856, 128.9363) centre (156.5871, 130.5398) ccw projected
  arc A419 (162.5856, 128.9363) -> (162.7525, 129.6961) centre (154.2966, 131.1558) ccw projected
  arc A420 (162.7525, 129.6961) -> (162.8835, 130.7559) centre (151.8305, 131.5838) ccw projected
  arc A421 (162.8835, 130.7559) -> (162.1949, 131.1285) centre (148.5, 105) ccw projected
  arc A422 (162.1949, 131.1285) -> (161.3793, 130.4392) centre (168.9335, 122.3281) ccw projected
  arc A423 (161.3793, 130.4392) -> (160.8346, 129.8839) centre (167.2263, 124.1586) ccw projected
  arc A424 (160.8346, 129.8839) -> (160.4936, 129.4687) centre (165.4579, 125.7392) ccw projected
  arc A425 (160.4936, 129.4687) -> (159.7632, 129.8134) centre (148.5, 105) ccw projected
  arc A426 (159.7632, 129.8134) -> (159.8669, 130.3405) centre (153.7284, 131.2744) ccw projected
  arc A427 (159.8669, 130.3405) -> (159.9492, 131.1141) centre (151.3841, 131.6347) ccw projected
  arc A428 (159.9492, 131.1141) -> (159.9628, 132.1819) centre (148.8858, 131.7888) ccw projected
  arc A429 (159.9628, 132.1819) -> (159.2375, 132.4765) centre (148.5, 105) ccw projected
  arc A430 (159.2375, 132.4765) -> (158.5026, 131.7016) centre (166.9032, 124.4708) ccw projected
  arc A431 (158.5026, 131.7016) -> (158.0223, 131.0897) centre (165.005, 126.1024) ccw projected
  arc A432 (158.0223, 131.0897) -> (157.729, 130.6396) centre (163.0734, 127.4788) ccw projected
  arc A433 (157.729, 130.6396) -> (156.9651, 130.9018) centre (148.5, 105) ccw projected
  arc A434 (156.9651, 130.9018) -> (157.0102, 131.4372) centre (150.8063, 131.6901) ccw projected
  arc A435 (157.0102, 131.4372) -> (157.007, 132.2151) centre (148.4365, 131.7903) ccw projected
  arc A436 (157.007, 132.2151) -> (156.903, 133.2779) centre (145.9365, 131.6687) ccw projected
  arc A437 (156.903, 133.2779) -> (156.1497, 133.4909) centre (148.5, 105) ccw projected
  arc A438 (156.1497, 133.4909) -> (155.5045, 132.6399) centre (164.6496, 126.3771) ccw projected
  arc A439 (155.5045, 132.6399) -> (155.0944, 131.9789) centre (162.5834, 127.79) ccw projected
  arc A440 (155.0944, 131.9789) -> (154.8525, 131.4992) centre (160.5121, 128.9456) ccw projected
  arc A441 (154.8525, 131.4992) -> (154.0644, 131.6758) centre (148.5, 105) ccw projected
  arc A442 (154.0644, 131.6758) -> (154.0503, 132.2129) centre (147.8561, 131.7819) ccw projected
  arc A443 (154.0503, 132.2129) -> (153.9615, 132.9857) centre (145.4898, 131.6208) ccw projected
  arc A444 (153.9615, 132.9857) -> (153.7412, 134.0307) centre (143.0183, 131.2248) ccw projected
  arc A445 (153.7412, 134.0307) -> (152.969, 134.1595) centre (148.5, 105) ccw projected
  arc A446 (152.969, 134.1595) -> (152.4214, 133.2427) centre (162.1999, 128.024) ccw projected
  arc A447 (152.4214, 133.2427) -> (152.0865, 132.5406) centre (159.9909, 129.201) ccw projected
  arc A448 (152.0865, 132.5406) -> (151.8988, 132.0372) centre (157.805, 130.1217) ccw projected
  arc A449 (151.8988, 132.0372) -> (151.096, 132.1261) centre (148.5, 105) ccw projected
  arc A450 (151.096, 132.1261) -> (151.023, 132.6583) centre (144.9138, 131.5485) ccw projected
  arc A451 (151.023, 132.6583) -> (150.8497, 133.4167) centre (142.5795, 131.128) ccw projected
  arc A452 (150.8497, 133.4167) -> (150.5158, 134.431) centre (140.1666, 130.4626) ccw projected
  arc A453 (150.5158, 134.431) -> (149.7341, 134.4742) centre (148.5, 105) ccw projected
  arc A454 (149.7341, 134.4742) -> (149.2907, 133.5027) centre (159.5839, 129.3913) ccw projected
  arc A455 (149.2907, 133.5027) -> (149.035, 132.768) centre (157.2588, 130.3182) ccw projected
  circle A456 centre (148.5, 105) radius 2.995
  arc A457 (149.6015, 112.7038) -> (149.519, 112.4481) centre (150.662, 112.2202) ccw
  arc A458 (150.2087, 113.6056) -> (149.6015, 112.7038) centre (152.6178, 111.3284) ccw
  arc A459 (152.528, 115.1478) -> (150.2087, 113.6056) centre (154.7109, 109.3498) ccw
  arc A460 (152.8274, 115.0238) -> (152.528, 115.1478) centre (148.5, 105) ccw
  arc A461 (153.3769, 112.2933) -> (152.8274, 115.0238) centre (147.184, 112.4675) ccw
  arc A462 (153.1685, 111.2263) -> (153.3769, 112.2933) centre (150.0631, 112.3865) ccw
  arc A463 (153.0461, 110.9871) -> (153.1685, 111.2263) centre (152.0767, 111.6342) ccw
  line L0 (152.4308, 110.1768) -> (153.0461, 110.9871)
  arc A464 (153.6768, 108.9308) -> (152.4308, 110.1768) centre (148.5, 105) ccw
  line L1 (154.4871, 109.5461) -> (153.6768, 108.9308)
  arc A465 (154.7263, 109.6685) -> (154.4871, 109.5461) centre (155.1342, 108.5767) ccw
  arc A466 (155.7933, 109.8769) -> (154.7263, 109.6685) centre (155.8865, 106.5631) ccw
  arc A467 (158.5238, 109.3274) -> (155.7933, 109.8769) centre (155.9675, 103.684) ccw
  arc A468 (158.6478, 109.028) -> (158.5238, 109.3274) centre (148.5, 105) ccw
  arc A469 (157.1056, 106.7087) -> (158.6478, 109.028) centre (152.8498, 111.2109) ccw
  arc A470 (156.2038, 106.1015) -> (157.1056, 106.7087) centre (154.8284, 109.1178) ccw
  arc A471 (155.9481, 106.019) -> (156.2038, 106.1015) centre (155.7202, 107.162) ccw
  line L2 (154.94, 105.8811) -> (155.9481, 106.019)
  arc A472 (154.94, 104.1189) -> (154.94, 105.8811) centre (148.5, 105) ccw
  line L3 (155.9481, 103.981) -> (154.94, 104.1189)
  arc A473 (156.2038, 103.8985) -> (155.9481, 103.981) centre (155.7202, 102.838) ccw
  arc A474 (157.1056, 103.2913) -> (156.2038, 103.8985) centre (154.8284, 100.8822) ccw
  arc A475 (158.6478, 100.972) -> (157.1056, 103.2913) centre (152.8498, 98.7891) ccw
  arc A476 (158.5238, 100.6726) -> (158.6478, 100.972) centre (148.5, 105) ccw
  arc A477 (155.7933, 100.1231) -> (158.5238, 100.6726) centre (155.9675, 106.316) ccw
  arc A478 (154.7263, 100.3315) -> (155.7933, 100.1231) centre (155.8865, 103.4369) ccw
  arc A479 (154.4871, 100.4539) -> (154.7263, 100.3315) centre (155.1342, 101.4233) ccw
  line L4 (153.6768, 101.0692) -> (154.4871, 100.4539)
  arc A480 (152.4308, 99.8232) -> (153.6768, 101.0692) centre (148.5, 105) ccw
  line L5 (153.0461, 99.0129) -> (152.4308, 99.8232)
  arc A481 (153.1685, 98.7737) -> (153.0461, 99.0129) centre (152.0767, 98.3658) ccw
  arc A482 (153.3769, 97.7067) -> (153.1685, 98.7737) centre (150.0631, 97.6135) ccw
  arc A483 (152.8274, 94.9762) -> (153.3769, 97.7067) centre (147.184, 97.5325) ccw
  arc A484 (152.528, 94.8522) -> (152.8274, 94.9762) centre (148.5, 105) ccw
  arc A485 (150.2087, 96.3944) -> (152.528, 94.8522) centre (154.7109, 100.6502) ccw
  arc A486 (149.6015, 97.2962) -> (150.2087, 96.3944) centre (152.6178, 98.6716) ccw
  arc A487 (149.519, 97.5519) -> (149.6015, 97.2962) centre (150.662, 97.7798) ccw
  line L6 (149.3811, 98.56) -> (149.519, 97.5519)
  arc A488 (147.6189, 98.56) -> (149.3811, 98.56) centre (148.5, 105) ccw
  line L7 (147.481, 97.5519) -> (147.6189, 98.56)
  arc A489 (147.3985, 97.2962) -> (147.481, 97.5519) centre (146.338, 97.7798) ccw
  arc A490 (146.7913, 96.3944) -> (147.3985, 97.2962) centre (144.3822, 98.6716) ccw
  arc A491 (144.472, 94.8522) -> (146.7913, 96.3944) centre (142.2891, 100.6502) ccw
  arc A492 (144.1726, 94.9762) -> (144.472, 94.8522) centre (148.5, 105) ccw
  arc A493 (143.6231, 97.7067) -> (144.1726, 94.9762) centre (149.816, 97.5325) ccw
  arc A494 (143.8315, 98.7737) -> (143.6231, 97.7067) centre (146.9369, 97.6135) ccw
  arc A495 (143.9539, 99.0129) -> (143.8315, 98.7737) centre (144.9233, 98.3658) ccw
  line L8 (144.5692, 99.8232) -> (143.9539, 99.0129)
  arc A496 (143.3232, 101.0692) -> (144.5692, 99.8232) centre (148.5, 105) ccw
  line L9 (142.5129, 100.4539) -> (143.3232, 101.0692)
  arc A497 (142.2737, 100.3315) -> (142.5129, 100.4539) centre (141.8658, 101.4233) ccw
  arc A498 (141.2067, 100.1231) -> (142.2737, 100.3315) centre (141.1135, 103.4369) ccw
  arc A499 (138.4762, 100.6726) -> (141.2067, 100.1231) centre (141.0325, 106.316) ccw
  arc A500 (138.3522, 100.972) -> (138.4762, 100.6726) centre (148.5, 105) ccw
  arc A501 (139.8944, 103.2913) -> (138.3522, 100.972) centre (144.1502, 98.7891) ccw
  arc A502 (140.7962, 103.8985) -> (139.8944, 103.2913) centre (142.1716, 100.8822) ccw
  arc A503 (141.0519, 103.981) -> (140.7962, 103.8985) centre (141.2798, 102.838) ccw
  line L10 (142.06, 104.1189) -> (141.0519, 103.981)
  arc A504 (142.06, 105.8811) -> (142.06, 104.1189) centre (148.5, 105) ccw
  line L11 (141.0519, 106.019) -> (142.06, 105.8811)
  arc A505 (140.7962, 106.1015) -> (141.0519, 106.019) centre (141.2798, 107.162) ccw
  arc A506 (139.8944, 106.7087) -> (140.7962, 106.1015) centre (142.1716, 109.1178) ccw
  arc A507 (138.3522, 109.028) -> (139.8944, 106.7087) centre (144.1502, 111.2109) ccw
  arc A508 (138.4762, 109.3274) -> (138.3522, 109.028) centre (148.5, 105) ccw
  arc A509 (141.2067, 109.8769) -> (138.4762, 109.3274) centre (141.0325, 103.684) ccw
  arc A510 (142.2737, 109.6685) -> (141.2067, 109.8769) centre (141.1135, 106.5631) ccw
  arc A511 (142.5129, 109.5461) -> (142.2737, 109.6685) centre (141.8658, 108.5767) ccw
  line L12 (143.3232, 108.9308) -> (142.5129, 109.5461)
  arc A512 (144.5692, 110.1768) -> (143.3232, 108.9308) centre (148.5, 105) ccw
  line L13 (143.9539, 110.9871) -> (144.5692, 110.1768)
  arc A513 (143.8315, 111.2263) -> (143.9539, 110.9871) centre (144.9233, 111.6342) ccw
  arc A514 (143.6231, 112.2933) -> (143.8315, 111.2263) centre (146.9369, 112.3865) ccw
  arc A515 (144.1726, 115.0238) -> (143.6231, 112.2933) centre (149.816, 112.4675) ccw
  arc A516 (144.472, 115.1478) -> (144.1726, 115.0238) centre (148.5, 105) ccw
  arc A517 (146.7913, 113.6056) -> (144.472, 115.1478) centre (142.2891, 109.3498) ccw
  arc A518 (147.3985, 112.7038) -> (146.7913, 113.6056) centre (144.3822, 111.3284) ccw
  arc A519 (147.481, 112.4481) -> (147.3985, 112.7038) centre (146.338, 112.2202) ccw
  line L14 (147.6189, 111.44) -> (147.481, 112.4481)
  arc A520 (149.3811, 111.44) -> (147.6189, 111.44) centre (148.5, 105) ccw
  line L15 (149.519, 112.4481) -> (149.3811, 111.44)
  circle A521 centre (148.5, 105) radius 2.995
  line L16 (140.0891, 100.3796) -> (142.099, 101.2121)
  arc A522 (144.7121, 98.599) -> (142.099, 101.2121) centre (142.8643, 99.3643) ccw
  line L17 (144.7121, 98.599) -> (143.8796, 96.5891)
  arc A523 (143.8796, 96.5891) -> (145.8197, 95.7854) centre (144.8496, 96.1872) ccw
  line L18 (145.8197, 95.7854) -> (146.6522, 97.7953)
  arc A524 (150.3478, 97.7953) -> (146.6522, 97.7953) centre (148.5, 97.03) ccw
  line L19 (150.3478, 97.7953) -> (151.1803, 95.7854)
  arc A525 (151.1803, 95.7854) -> (153.1204, 96.5891) centre (152.1504, 96.1872) ccw
  line L20 (153.1204, 96.5891) -> (152.2879, 98.599)
  arc A526 (154.901, 101.2121) -> (152.2879, 98.599) centre (154.1357, 99.3643) ccw
  line L21 (154.901, 101.2121) -> (156.9109, 100.3796)
  arc A527 (156.9109, 100.3796) -> (157.7146, 102.3197) centre (157.3128, 101.3496) ccw
  line L22 (157.7146, 102.3197) -> (155.7047, 103.1522)
  arc A528 (155.7047, 106.8478) -> (155.7047, 103.1522) centre (156.47, 105) ccw
  line L23 (155.7047, 106.8478) -> (157.7146, 107.6803)
  arc A529 (157.7146, 107.6803) -> (156.9109, 109.6204) centre (157.3128, 108.6504) ccw
  line L24 (156.9109, 109.6204) -> (154.901, 108.7879)
  arc A530 (152.2879, 111.401) -> (154.901, 108.7879) centre (154.1357, 110.6357) ccw
  line L25 (152.2879, 111.401) -> (153.1204, 113.4109)
  arc A531 (153.1204, 113.4109) -> (151.1803, 114.2146) centre (152.1504, 113.8128) ccw
  line L26 (151.1803, 114.2146) -> (150.3478, 112.2047)
  arc A532 (146.6522, 112.2047) -> (150.3478, 112.2047) centre (148.5, 112.97) ccw
  line L27 (146.6522, 112.2047) -> (145.8197, 114.2146)
  arc A533 (145.8197, 114.2146) -> (143.8796, 113.4109) centre (144.8496, 113.8128) ccw
  line L28 (143.8796, 113.4109) -> (144.7121, 111.401)
  arc A534 (142.099, 108.7879) -> (144.7121, 111.401) centre (142.8643, 110.6357) ccw
  line L29 (142.099, 108.7879) -> (140.0891, 109.6204)
  arc A535 (140.0891, 109.6204) -> (139.2854, 107.6803) centre (139.6872, 108.6504) ccw
  line L30 (139.2854, 107.6803) -> (141.2953, 106.8478)
  arc A536 (141.2953, 103.1522) -> (141.2953, 106.8478) centre (140.53, 105) ccw
  line L31 (141.2953, 103.1522) -> (139.2854, 102.3197)
  arc A537 (139.2854, 102.3197) -> (140.0891, 100.3796) centre (139.6872, 101.3496) ccw
  point P0 (0, 0)
  point P1 (0, 0)
  constraints: 160 point on circle, 82 centre point, 64 end point
extrude "押し出し2" cut sketch "スケッチ2" against normal blind 4 contours A456 | A531 L25 A530 L24 A529 L23 A528 L22 A527 L21 A526 L20 A525 L19 A524 L18 A523 L17 A522 L16 A537 L31 A536 L30 A535 L29 A534 L28 A533 L27 A532 L26